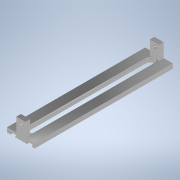
# Autodesk Inventor part: base plate
Saved by Autodesk Inventor 2020 (Build 240168000, 168)
## iProperties
Created: 2020-07-02
Part Number: base plate
Material: Generic
Document SubType Name: Modeling
Designer: Ashiqrahman
Density: 1 g/cm^3
Appearance: Chrome - Polished
Author: Ashiqrahman
Autodesk Inventor part; units mm, degrees
ref_plane "YZ Plane" through (0, 0, 0) normal (1, 0, 0) x (0, 1, 0)
ref_plane "XZ Plane" through (0, 0, 0) normal (0, 1, 0) x (-1, 0, 0)
ref_plane "XY Plane" through (0, 0, 0) normal (0, 0, 1) x (1, 0, 0)
sketch "Sketch1" plane through (0, 0, 0) normal (0, 1, 0) x (-1, 0, 0)
  line L0 (-30, -150) -> (30, -150)
  line L1 (30, -150) -> (30, 150)
  line L2 (30, 150) -> (-30, 150)
  line L3 (-30, 150) -> (-30, -150)
  line L4 (-30, -150) -> (30, 150) construction
  line L5 (30, -150) -> (-30, 150) construction
  point P0 (0, 0)
  dimension "d0" = 60
  dimension "d1" = 300
  constraints: 12 end point, 2 midpoint, 2 parallel, 1 horizontal, 1 perpendicular
  measures "d0" distance of L2.end L1.end
  measures "d1" distance of L1.end L0.end
extrude "Extrusion1" add sketch "Sketch1" along normal blind 10
sketch "Sketch2" plane through (-30, 0, 150) normal (0, 0, 1) x (1, 0, 0)
  line L0 (4.1132, -5) -> (19.8868, -5)
  line L1 (19.8868, -5) -> (19.8868, 5)
  line L2 (19.8868, 5) -> (4.1132, 5)
  line L3 (4.1132, 5) -> (4.1132, -5)
  line L4 (4.1132, -5) -> (19.8868, 5) construction
  line L5 (19.8868, -5) -> (4.1132, 5) construction
  line L6 (4.1132, 5) -> (7, 0)
  line L7 (0, 0) -> (60, 0) projected
  line L8 (12, 0) -> (12, 10) construction
  line L9 (19.8868, 5) -> (17, 0)
  line L10 (7, 0) -> (4.1132, 0)
  line L11 (17, 0) -> (19.8868, 0)
  line L12 (30, 0) -> (30, 10)
  line L13 (0, 10) -> (60, 10) projected
  line L14 (40.1132, -5) -> (40.1132, 5)
  line L15 (40.1132, 5) -> (55.8868, 5)
  line L16 (55.8868, 5) -> (55.8868, -5)
  line L17 (55.8868, 5) -> (53, 0)
  line L18 (40.1132, 5) -> (43, 0)
  line L19 (53, 0) -> (55.8868, 0)
  line L20 (43, 0) -> (40.1132, 0)
  line L21 (43, 0) -> (53, 0)
  line L22 (7, 0) -> (17, 0)
  point P0 (17, 0)
  dimension "d5" = 10
  dimension "d6" = 10
  dimension "d7" = 60
  dimension "d10" = 12
  constraints: 42 end point, 9 symmetric about line, 8 midpoint, 3 point on line, 2 parallel, 1 collinear, 1 horizontal, 1 perpendicular, 1 vertical
  measures "d5" distance of L1.end L0.end
  measures "d6" distance of L9.end L6.end
  measures "d7" angle of L6 L2
  measures "d10" distance of L7.start L8.start
extrude "Extrusion2" cut sketch "Sketch2" against normal up to surface (300 mm away) contours L2 L9 L7 L6
pattern_linear "Rectangular Pattern1" count 2 spacing 36 along (1, 0, 0) of "Extrusion2"
sketch "Sketch3" plane through (0, 10, 0) normal (0, 1, 0) x (1, 0, 0)
  line L0 (0, 130) -> (0, -130) construction
  line L1 (10.1132, -150) -> (10.1132, 150) projected
  line L2 (-8, 130) -> (-8, -130)
  line L3 (8, -130) -> (8, 130)
  arc A0 (8, 130) -> (-8, 130) centre (0, 130) ccw
  arc A1 (-8, -130) -> (8, -130) centre (0, -130) ccw
  point P0 (0, 0)
  dimension "d14" = 260
  dimension "d15" = 8
  constraints: 8 end point, 4 point on circle, 4 tangent, 2 centre point, 2 parallel, 1 midpoint
  measures "d14" distance of L2.start L2.end
  measures "d15" radius of A0
extrude "Extrusion3" cut sketch "Sketch3" against normal through all
sketch "Sketch4" plane through (0, 10, 0) normal (0, 1, 0) x (1, 0, 0)
  line L0 (-30, 150) -> (-30, -150) projected
  line L1 (-30, -150) -> (-10, -150)
  line L2 (-10, -150) -> (-10, -140)
  line L3 (-10, -140) -> (-30, -140)
  line L4 (-30, -140) -> (-30, -150)
  line L5 (30, 150) -> (-30, 150) projected
  line L6 (30, 150) -> (10, 150)
  line L7 (10, 150) -> (10, 140)
  line L8 (10, 140) -> (30, 140)
  line L9 (30, 140) -> (30, 150)
  line L10 (-30, 0) -> (-10, 0)
  line L11 (-10, 0) -> (-10, -10)
  line L12 (-10, -10) -> (-30, -10)
  line L13 (-30, -10) -> (-30, 0)
  line L14 (30, -150) -> (30, 150) projected
  line L15 (30, 0) -> (10, 0)
  line L16 (10, 0) -> (10, -10)
  line L17 (10, -10) -> (30, -10)
  line L18 (30, -10) -> (30, 0)
  point P0 (0, 0)
  dimension "d18" = 20
  dimension "d19" = 10
  dimension "d20" = 20
  dimension "d21" = 10
  dimension "d22" = 20
  dimension "d23" = 10
  dimension "d24" = 20
  dimension "d25" = 10
  constraints: 32 end point, 8 parallel, 4 horizontal, 4 perpendicular, 2 midpoint
  measures "d18" distance of L3.end L2.end
  measures "d19" distance of L2.end L1.end
  measures "d20" distance of L8.end L7.end
  measures "d21" distance of L7.end L6.end
  measures "d22" distance of L11.end L12.end
  measures "d23" distance of L10.end L11.end
  measures "d24" distance of L17.end L16.end
  measures "d25" distance of L16.end L15.end
extrude "Extrusion4" add sketch "Sketch4" along normal blind 30
sketch "Sketch5" plane through (30, 0, 150) normal (0, 0, 1) x (1, 0, 0)
  line L0 (-60, 40) -> (-40, 40) projected
  line L1 (-40, 10) -> (-40, 40) projected
  line L2 (-60, 40) -> (-40, 40)
  line L3 (-40, 40) -> (-40, 10)
  line L4 (-40, 10) -> (-60, 10)
  line L5 (-60, 10) -> (-60, 40)
  circle A0 centre (-50, 32) radius 4
  point P0 (-30, 0)
  dimension "d28" = 8
  dimension "d36" = 8
  constraints: 8 end point, 2 parallel, 1 centre point, 1 horizontal, 1 perpendicular
  measures "d28" diameter of A0
  measures "d36" distance from line of L0 A0.centre
extrude "Extrusion5" cut sketch "Sketch5" against normal through all contours A0
sketch "Sketch6" plane through (-30, 0, -150) normal (0, 0, -1) x (-1, 0, 0)
  line L0 (-60, 40) -> (-40, 40) projected
  line L1 (-40, 10) -> (-60, 10) projected
  line L2 (-60, 40) -> (-40, 40)
  line L3 (-40, 40) -> (-40, 10)
  line L4 (-40, 10) -> (-60, 10)
  line L5 (-60, 10) -> (-60, 40)
  circle A0 centre (-50, 32) radius 4
  point P0 (-30, 0)
  dimension "d31" = 8
  dimension "d35" = 8
  constraints: 8 end point, 2 parallel, 1 centre point, 1 horizontal, 1 perpendicular
  measures "d31" diameter of A0
  measures "d35" distance from line of L0 A0.centre
extrude "Extrusion6" cut sketch "Sketch6" against normal through all contours A0
fillet "Fillet1" radius 2 16 edges at (-8, 0, 0) (0, 0, 138) (8, 0, 0) (0, 0, -138) (24, 32, 10) (-24, 32, 0) (-24, 32, 10) (0, 10, 138) (-8, 10, 0) (0, 10, -138) (8, 10, 0) (24, 32, 0) (24, 32, -140) (24, 32, -150) (-24, 32, 150) (-24, 32, 140)
body "Solid1"
